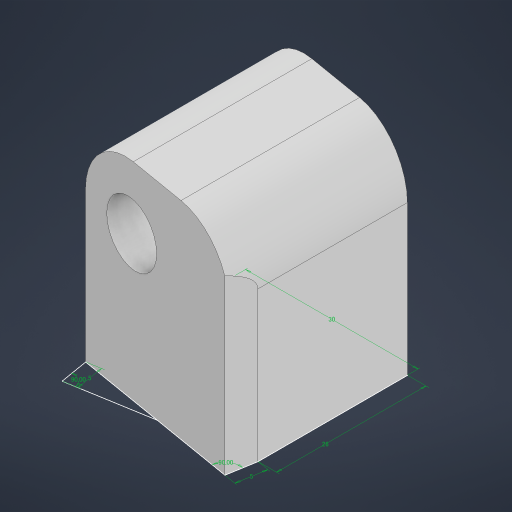
# Autodesk Inventor part: default
Saved by Autodesk Inventor 2024.3 (Build 283343000, 343)
## iProperties
Created: 2024-07-26
Part Number: default
Material: 一般
Document SubType Name: Modeling
Designer: ktamu
Density: 1 g/cm^3
Appearance: 既定
Author: ktamu
Autodesk Inventor part; units mm, degrees
ref_plane "YZ Plane" through (0, 0, 0) normal (1, 0, 0) x (0, 1, 0)
ref_plane "XZ Plane" through (0, 0, 0) normal (0, 1, 0) x (-1, 0, 0)
ref_plane "XY Plane" through (0, 0, 0) normal (0, 0, 1) x (1, 0, 0)
sketch "BaseSC" plane through (0, 0, 0) normal (0, 1, 0) x (-1, 0, 0)
  line L0 (15, 13) -> (-15, 13)
  line L1 (-15, 13) -> (-15, -13)
  line L2 (-15, -13) -> (15, -13)
  line L3 (15, -13) -> (15, 13)
  line L4 (15, 13) -> (-15, -13) construction
  line L5 (-15, 13) -> (15, -13) construction
  line L6 (15, 13) -> (14.1667, 17.9301)
  line L7 (14.1667, 17.9301) -> (-15, 13)
  line L8 (0, 0) -> (8.3423, 0)
  line L9 (15, -13) -> (14.1667, -17.9301)
  line L10 (14.1667, -17.9301) -> (-15, -13)
  line L11 (-15, 13) -> (-14.1667, 17.9301)
  line L12 (-14.1667, 17.9301) -> (15, 13)
  dimension "d0" = 30
  dimension "d1" = 26
  dimension "d9" = 5
  dimension "d10" = 90
  dimension "d17" = 5
  dimension "d18" = 90
  constraints: 26 end point, 2 horizontal, 2 midpoint, 2 parallel, 1 perpendicular, 1 symmetric about line
  measures "d0" distance of L2.end L1.end
  measures "d1" distance of L0.end L1.end
  measures "d9" distance of L0.start L6.end
  measures "d10" angle of L7 L6
  measures "d17" distance of L0.end L11.end
  measures "d18" angle of L12 L11
sketch "スケッチ2" plane through (0, 0, 0) normal (0, 0, 1) x (1, 0, 0)
  point P0 (0, 0)
extrude "押し出し1" add sketch "BaseSC" against normal blind 30 contours L3 L2 L1 L0
sketch "スケッチ3" plane through (15, 0, 13) normal (1, 0, 0) x (0, 0, -1)
  line L0 (2.5, -1.5742) -> (23.5, -1.5742)
  line L1 (23.5, -1.5742) -> (23.5, -28.5742)
  line L2 (23.5, -28.5742) -> (2.5, -28.5742)
  line L3 (2.5, -28.5742) -> (2.5, -1.5742)
  line L4 (2.5, -1.5742) -> (23.5, -28.5742) construction
  line L5 (23.5, -1.5742) -> (2.5, -28.5742) construction
  ellipse E0 centre (13, -15.0742) end of major axis (23.5, -15.0742) minor radius 13.5
  point P0 (13, 0)
  dimension "d5" = 21
  dimension "d6" = 27
  constraints: 12 end point, 2 midpoint, 2 parallel, 1 centre point, 1 coincident, 1 horizontal, 1 perpendicular
  measures "d5" distance of L1.end L2.end
  measures "d6" distance of L0.end L1.end
extrude "押し出し2" cut sketch "スケッチ3" against normal through all contours E0
extrude "押し出し3" add sketch "BaseSC" along normal blind 36 contours L3 L2 L1 L0 | L9 L10 L2
extrude "押し出し5" add sketch "BaseSC" along normal blind 36 contours L0 L7 L12 | L11 L12 L7
sketch "スケッチ5" plane through (-14.1667, 0, -17.9301) normal (0.1666667, 0, -0.9860133) x (-0.9860133, 0, -0.1666667)
  circle A0 centre (-14.1422, 25) radius 5.3
  line L0 (-29.5804, 0) -> (0, 0) projected
  point P0 (-16.9569, 0)
  dimension "d21" = 10.6
  dimension "d22" = 25
  constraints: 1 centre point
  measures "d21" diameter of A0
  measures "d22" distance from line of L0 A0.centre
extrude "押し出し6" cut sketch "スケッチ5" against normal through all
sketch "スケッチ6" plane through (0, -30, 0) normal (0, -1, 0) x (1, 0, 0)
  line L0 (15, -1) -> (-15, -1)
  line L1 (-15, -1) -> (-15, 1)
  line L2 (-15, 1) -> (15, 1)
  line L3 (15, 1) -> (15, -1)
  line L4 (15, -1) -> (-15, 1) construction
  line L5 (-15, -1) -> (15, 1) construction
  point P0 (0, 0)
  dimension "d25" = 30
  dimension "d26" = 2
  constraints: 12 end point, 2 midpoint, 2 parallel, 1 horizontal, 1 perpendicular
  measures "d25" distance of L1.end L2.end
  measures "d26" distance of L0.end L1.end
extrude "押し出し7" cut sketch "スケッチ6" against normal blind 5
fillet "フィレット1" radius 10 2 edges at (15, 36, 0) (-15, 36, 0)
sketch "スケッチ7" plane through (-15, -30, 13) normal (0, 0, 1) x (1, 0, 0)
  line L0 (30, 30) -> (0, 30) projected
  line L1 (0, 0) -> (0, 30) projected
  line L2 (30, 0) -> (0, 0) projected
  line L3 (30, 30) -> (30, 0) projected
  point P0 (15, 30)
extrude "押し出し8" cut sketch "スケッチ7" against normal through all
